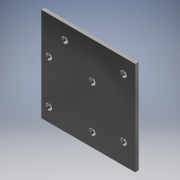
# Autodesk Inventor part: Steel Bracing
Saved by Autodesk Inventor 2019.4 (Build 234330000, 330)
## iProperties
Created: 2020-01-10
Part Number: Steel Bracing
Material: Steel, Alloy
Document SubType Name: Modeling
Designer: Mark
Mass: 143.685 g
Surface Area: 137.525 cm^2
Volume: 18.588 cm^3
Density: 7.73 g/cm^3
Appearance: Semi-Polished
Author: Mark
Autodesk Inventor part; units mm, degrees
ref_plane "YZ Plane" through (0, 0, 0) normal (1, 0, 0) x (0, 1, 0)
ref_plane "XZ Plane" through (0, 0, 0) normal (0, 1, 0) x (-1, 0, 0)
ref_plane "XY Plane" through (0, 0, 0) normal (0, 0, 1) x (1, 0, 0)
sketch "Sketch1" plane through (0, 0, 0) normal (0, 0, 1) x (1, 0, 0)
  line L0 (0, 0) -> (80, 0)
  line L1 (80, 0) -> (80, 80)
  line L2 (80, 80) -> (0, 80)
  line L3 (0, 80) -> (0, 0)
  dimension "d0" = 80
  dimension "d1" = 80
  constraints: 8 end point, 2 parallel, 1 horizontal, 1 perpendicular
  measures "d0" distance of L2.end L1.end
  measures "d1" distance of L1.end L0.end
extrude "Extrusion1" add sketch "Sketch1" along normal blind 3
sketch "Sketch2" plane through (0, 0, 3) normal (0, 0, 1) x (1, 0, 0)
  circle A0 centre (20, 67.5) radius 2.75
  circle A1 centre (70, 67.5) radius 2.75
  line L0 (80, 80) -> (0, 80) projected
  line L1 (80, 0) -> (80, 80) projected
  circle A2 centre (70, 17.5) radius 2.75
  point P0 (0, 0)
  dimension "d4" = 5.5
  dimension "d5" = 5.5
  dimension "d6" = 12.5
  dimension "d7" = 10
  dimension "d8" = 50
  dimension "d9" = 12.5
  dimension "d10" = 5.5
  dimension "d11" = 50
  dimension "d12" = 10
  constraints: 3 centre point
  measures "d4" diameter of A0
  measures "d5" diameter of A1
  measures "d6" distance from line of L0 A1.centre
  measures "d7" distance from line of L1 A1.centre
  measures "d8" distance of A1.centre A0.centre
  measures "d9" distance from line of L0 A0.centre
  measures "d10" diameter of A2
  measures "d11" distance between centres of A1 A2
  measures "d12" distance from line of L1 A2.centre
extrude "Extrusion2" cut sketch "Sketch2" against normal blind 3
sketch "Sketch3" plane through (0, 0, 3) normal (0, 0, 1) x (1, 0, 0)
  circle A0 centre (6.5, 48.5) radius 3.25
  circle A1 centre (43.5, 48.5) radius 3.25
  circle A2 centre (43.5, 11.5) radius 3.25
  circle A3 centre (6.5, 11.5) radius 3.25
  line L0 (0, 80) -> (0, 0) projected
  line L1 (0, 0) -> (80, 0) projected
  dimension "d15" = 6.5
  dimension "d16" = 6.5
  dimension "d17" = 6.5
  dimension "d18" = 6.5
  dimension "d19" = 37
  dimension "d20" = 37
  dimension "d21" = 37
  dimension "d22" = 37
  dimension "d23" = 37
  dimension "d24" = 37
  dimension "d25" = 6.5
  dimension "d26" = 11.5
  constraints: 4 centre point
  measures "d15" diameter of A0
  measures "d16" diameter of A1
  measures "d17" diameter of A2
  measures "d18" diameter of A3
  measures "d19" distance of A2.centre A3.centre
  measures "d20" horizontal distance of A1.centre A3.centre
  measures "d21" distance of A3.centre A0.centre
  measures "d22" distance of A1.centre A2.centre
  measures "d23" horizontal distance of A0.centre A2.centre
  measures "d24" distance of A0.centre A1.centre
  measures "d25" distance from line of L0 A3.centre
  measures "d26" distance from line of L1 A3.centre
extrude "Extrusion3" cut sketch "Sketch3" against normal blind 10
body "Solid1"
